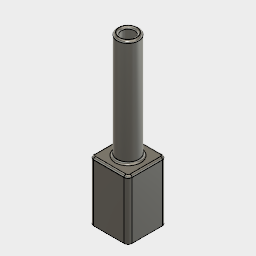
GatorGripAdapter v2 (Autodesk Fusion 360 design; units mm, degrees)
Autodesk Fusion 360 part; units mm, degrees
sketch "Sketch1" plane through (0, 0, 0) normal (0, 1, 0) x (1, 0, 0)
  line L0 (4.875, 4.875) -> (-4.875, 4.875)
  line L1 (-4.875, 4.875) -> (-4.875, -4.875)
  line L2 (-4.875, -4.875) -> (4.875, -4.875)
  line L3 (4.875, -4.875) -> (4.875, 4.875)
  line L4 (4.875, 4.875) -> (-4.875, -4.875) construction
  line L5 (-4.875, 4.875) -> (4.875, -4.875) construction
  circle A0 centre (0, 0) radius 2.75
  circle A1 centre (0, 0) radius 1.7
  dimension "d1" = 9.75
  dimension "d2" = 9.75
  dimension "d3" = 5.5
  dimension "d4" = 3.4
  constraint perpendicular L0 L1
  constraint parallel L0 L2
  constraint parallel L1 L3
  constraint horizontal L0
  constraint coincident L4
  constraint coincident L5
  constraint concentric A0 A1
  measures "d3" diameter of A0
  measures "d4" diameter of A1
extrude "Extrude1" add sketch "Sketch1" along normal blind 42 contours A0
extrude "Extrude2" add sketch "Sketch1" along normal blind 15 contours L0 L1 L2 L3
fillet "Fillet1" radius 1 4 edges at (4.875, 7.5, 4.875) (4.875, 7.5, -4.875) (-4.875, 7.5, 4.875) (-4.875, 7.5, -4.875)
fillet "Fillet2" radius 0.5 8 edges at (-4.5821, 15, 4.5821) (0, 15, 4.875) (4.5821, 15, 4.5821) (4.875, 15, 0) (4.5821, 15, -4.5821) (0, 15, -4.875) (-4.5821, 15, -4.5821) (-4.875, 15, 0)
fillet "Fillet3" radius 0.5 1 edges at (-2.5639, 15, 0.9944)
fillet "Fillet4" radius 0.5 2 edges at (-2.5639, 42, 0.9944) (-1.585, 42, -0.6147)
extrude "Extrude3" add sketch "Sketch1" along normal blind 30 contours A1
